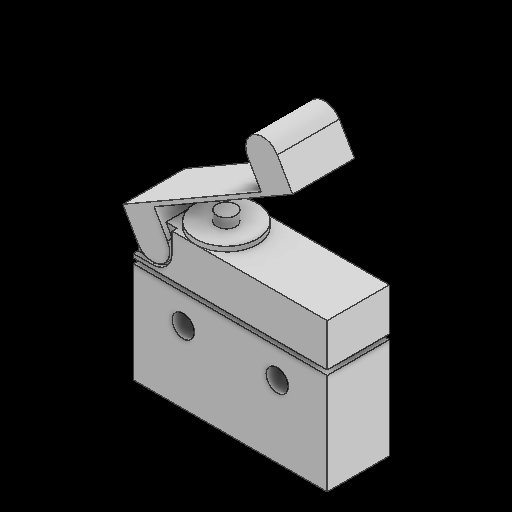
# Autodesk Inventor part: ArmLimitSwitch
Saved by Autodesk Inventor 2025.2 (Build 292293000, 293)
## iProperties
Created: 2026-03-16
Part Number: ArmLimitSwitch
Material: Generic
Document SubType Name: Modeling
Designer: valer
Density: 1 g/cm^3
Appearance: Default
Author: valer
Autodesk Inventor part; units mm, degrees
ref_plane "YZ Plane" through (0, 0, 0) normal (1, 0, 0) x (0, 1, 0)
ref_plane "XZ Plane" through (0, 0, 0) normal (0, 1, 0) x (-1, 0, 0)
sketch "LimitSwitchBody" plane through (0, 0, 0) normal (0, 0, 1) x (1, 0, 0)
  line L0 (-10, -7.65) -> (10, -7.65)
  line L1 (10, -7.65) -> (10, 7.65)
  line L2 (10, 7.65) -> (-10, 7.65)
  line L3 (-10, 7.65) -> (-10, -7.65)
  line L4 (-10, -7.65) -> (10, 7.65) construction
  line L5 (10, -7.65) -> (-10, 7.65) construction
  line L6 (-10, -0.25) -> (10, -0.25) construction
  circle A0 centre (4.85, -0.25) radius 1.15
  line L7 (3.7, -1.4) -> (6, -1.4) construction
  line L8 (6, -1.4) -> (6, 0.9) construction
  line L9 (6, 0.9) -> (3.7, 0.9) construction
  line L10 (3.7, 0.9) -> (3.7, -1.4) construction
  line L11 (3.7, -1.4) -> (6, 0.9) construction
  line L12 (6, -1.4) -> (3.7, 0.9) construction
  line L13 (0, -10.71) -> (0, 10.71) construction
  circle A1 centre (-4.85, -0.25) radius 1.15
  point P0 (0, 0)
  dimension "d0" = 20
  dimension "d1" = 15.3
  dimension "d2" = 2.3
  dimension "d3" = 4
  dimension "d4" = 7.4
  constraints: 26 end point, 4 midpoint, 4 parallel, 3 perpendicular, 3 point on line, 2 centre point, 2 horizontal, 2 tangent, 1 symmetric about line, 1 other
  measures "d0" distance of L1.end L2.end
  measures "d1" distance of L0.end L1.end
  measures "d2" diameter of A0
  measures "d3" distance between parallel lines of L1 L8
  measures "d4" distance from line of L0 A0.centre
extrude "LimitSwitchBodyFeature" add sketch "LimitSwitchBody" along normal mid plane 6.4
ref_plane "EtchPlane" through (-10, 3.25, -3.2) normal (0, 1, 0) x (1, 0, 0)
sketch "EtchProfile" plane through (-10, 3.25, -3.2) normal (0, 1, 0) x (1, 0, 0)
  line L0 (0, 0) -> (20, 0) projected
  line L1 (0, 0) -> (0, -6.4) projected
  line L2 (20, -6.4) -> (0, -6.4) projected
  line L3 (20, 0) -> (20, -6.4) projected
  line L4 (0.5, -5.9) -> (0.5, 0.5)
  line L5 (0.5, 0.5) -> (19.5, 0.5)
  line L6 (19.5, 0.5) -> (19.5, -5.9)
  line L7 (19.5, -5.9) -> (0.5, -5.9)
  point P0 (10, -3.2)
  dimension "d8" = 0.5
  constraints: 8 end point, 3 other
  measures "d8" distance between parallel lines of L2 L7
extrude "EtchFeature" cut sketch "EtchProfile" against normal blind 0.5 contours L0 L4 L7 L6 L3 L2 L1
sketch "HingeIndent" plane through (0, 0, 3.2) normal (0, 0, 1) x (1, 0, 0)
  line L0 (-10, 7.65) -> (-10, 3.25) projected
  line L1 (-10, 7.65) -> (-6, 7.65)
  line L2 (-6, 7.65) -> (-6, 3.65)
  line L3 (-6, 3.65) -> (-10, 3.65)
  line L4 (-10, 3.65) -> (-10, 7.65)
  circle A0 centre (-8, 5.65) radius 2
  point P0 (0, 0)
  point P1 (-8, 3.65)
  point P2 (-6, 5.65)
  dimension "d11" = 4
  constraints: 8 end point, 3 tangent, 2 parallel, 2 perpendicular, 1 centre point, 1 horizontal
  measures "d11" distance of L2.end L3.end
extrude "HingeIndentFeature" cut sketch "HingeIndent" against normal blind 0.5 contours L1 A0 L0 | A0 L3 L0 | A0 | L1 L2 A0
mirror "HingeMirrorFeature" about plane through (0, 0, 0) normal (0, 0, 1) of "HingeIndentFeature"
sketch "ButtonHousing" plane through (10, 7.65, 3.2) normal (0, 1, 0) x (1, 0, 0)
  line L0 (-24, 3.2) -> (4, 3.2) construction
  line L1 (-20, 5.9) -> (-20, 0.5) construction
  circle A0 centre (-13.6, 3.2) radius 3.2
  line L2 (0, 0) -> (-16, 0) projected
  point P0 (-10, 3.2)
  dimension "d14" = 6.4
  constraints: 1 centre point, 1 point on line, 1 tangent
  measures "d14" distance from line of A0.centre L1
extrude "ButtonHousingFeature" add sketch "ButtonHousing" along normal blind 0.5
sketch "Button" plane through (-3.6, 8.15, 0) normal (0, 1, 0) x (1, 0, 0)
  circle A0 centre (0, 0) radius 3.2 construction
  circle A1 centre (0, 0) radius 1
  point P0 (3.6, 0)
  dimension "d17" = 2
  constraints: 1 centre point, 1 coincident
  measures "d17" diameter of A1
extrude "ButtonFeature" add sketch "Button" along normal blind 1
sketch "Lever" plane through (0, 0, 2.7) normal (0, 0, 1) x (1, 0, 0)
  arc A0 (-8, 3.65) -> (-6, 5.65) centre (-8, 5.65) ccw projected
  circle A1 centre (-8, 5.65) radius 1.75
  line L0 (-9.5155, 4.775) -> (-10.8905, 7.1566)
  line L1 (-10.8905, 7.1566) -> (-7.8595, 8.9066)
  line L2 (-7.8595, 8.9066) -> (-6.4845, 6.525)
  line L3 (-9.375, 8.0316) -> (-8, 5.65) construction
  line L4 (-10, 3.25) -> (10, 3.25) projected
  line L5 (-7.8595, 8.9066) -> (6.43, 17.1566)
  line L6 (-10.8905, 7.1566) -> (-11.0905, 7.503)
  line L7 (-11.0905, 7.503) -> (6.23, 17.503)
  line L8 (6.23, 17.503) -> (6.43, 17.1566)
  line L9 (-2.4303, 12.503) -> (-2.2303, 12.1566) construction
  circle A2 centre (3.3394, 19.0095) radius 1.75
  line L10 (6.23, 17.503) -> (4.855, 19.8845)
  line L11 (1.8239, 18.1345) -> (3.1989, 15.753)
  point P0 (0, 0)
  dimension "d20" = 0.25
  dimension "d21" = 2.75
  dimension "d22" = 3.5
  dimension "d23" = 120
  dimension "d24" = 20
  dimension "d25" = 0.4
  constraints: 22 end point, 8 perpendicular, 4 point on circle, 4 tangent, 3 point on line, 2 centre point, 2 midpoint, 1 coincident, 1 equal radius, 1 parallel
  measures "d20" radial gap between concentric circles of A0 A1
  measures "d21" distance from line of L1 L3.end
  measures "d22" diameter of A1
  measures "d23" angle of L4 L3
  measures "d24" distance of L6.end L7.end
  measures "d25" distance between parallel lines of L5 L7
extrude "LeverFeature" add sketch "Lever" along normal up to surface (0.5 mm away)
mirror "LeverMirrorFeature" about plane through (0, 0, 0) normal (0, 0, 1) of "LeverFeature"
sketch "LeverConnect" plane through (0, 0, 2.7) normal (0, 0, -1) x (-1, 0, 0)
  line L0 (10, 5.6141) -> (10, 7.65) projected
  line L1 (11.0905, 7.503) -> (10, 5.6141) projected
  line L2 (-3.1989, 15.753) -> (11.0905, 7.503) projected
  line L3 (-1.8239, 18.1345) -> (-3.1989, 15.753) projected
  arc A0 (-1.8239, 18.1345) -> (-4.855, 19.8845) centre (-3.3394, 19.0095) ccw projected
  line L4 (-6.43, 17.1566) -> (-4.855, 19.8845) projected
  line L5 (7.8595, 8.9066) -> (-6.43, 17.1566) projected
  line L6 (7.134, 7.65) -> (7.8595, 8.9066) projected
  line L7 (10, 7.65) -> (7.134, 7.65) projected
  point P0 (0, 0)
extrude "LeverConnectFeature" add sketch "LeverConnect" along normal up to surface (5.4 mm away)
equation "\"d26\" = d25"
body "Solid1"
